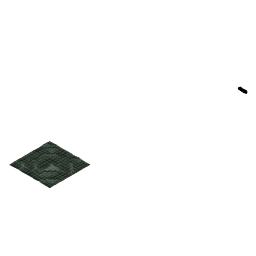
portal (Autodesk Fusion 360 design; units mm, degrees)
Autodesk Fusion 360 part; units mm, degrees
sketch "Sketch1" plane through (0, 0, 0) normal (0, 0, 1) x (1, 0, 0)
  line L0 (0, 0) -> (-55.5557, 0)
  line L1 (-55.5557, 0) -> (-55.5557, 55.5557)
  line L2 (-55.5557, 55.5557) -> (0, 55.5557)
  line L3 (0, 55.5557) -> (0, 0)
  line L4 (-55.5557, 55.5557) -> (0, 55.5557)
  line L5 (0, 55.5557) -> (0, 111.1113)
  line L6 (0, 111.1113) -> (-55.5557, 111.1113)
  line L7 (-55.5557, 111.1113) -> (-55.5557, 55.5557)
  line L8 (-55.5557, 111.1113) -> (0, 111.1113)
  line L9 (0, 111.1113) -> (0, 166.667)
  line L10 (0, 166.667) -> (-55.5557, 166.667)
  line L11 (-55.5557, 166.667) -> (-55.5557, 111.1113)
  line L12 (-55.5557, 166.667) -> (0, 166.667)
  line L13 (0, 166.667) -> (0, 222.2227)
  line L14 (0, 222.2227) -> (-55.5557, 222.2227)
  line L15 (-55.5557, 222.2227) -> (-55.5557, 166.667)
  line L16 (-55.5557, 0) -> (0, 0)
  line L17 (0, 0) -> (0, -55.5557)
  line L18 (0, -55.5557) -> (-55.5557, -55.5557)
  line L19 (-55.5557, -55.5557) -> (-55.5557, 0)
  line L20 (0, 0) -> (55.5557, 0)
  line L21 (55.5557, 0) -> (55.5557, -55.5557)
  line L22 (55.5557, -55.5557) -> (0, -55.5557)
  line L23 (0, -55.5557) -> (0, 0)
  line L24 (55.5557, 0) -> (111.1113, 0)
  line L25 (111.1113, 0) -> (111.1113, -55.5557)
  line L26 (111.1113, -55.5557) -> (55.5557, -55.5557)
  line L27 (55.5557, -55.5557) -> (55.5557, 0)
  line L28 (111.1113, -55.5557) -> (166.667, -55.5557)
  line L29 (166.667, -55.5557) -> (166.667, 0)
  line L30 (166.667, 0) -> (111.1113, 0)
  line L31 (111.1113, 0) -> (111.1113, -55.5557)
  line L32 (166.667, 0) -> (111.1113, 0)
  line L33 (111.1113, 0) -> (111.1113, 55.5557)
  line L34 (111.1113, 55.5557) -> (166.667, 55.5557)
  line L35 (166.667, 55.5557) -> (166.667, 0)
  line L36 (111.1113, 55.5557) -> (166.667, 55.5557)
  line L37 (166.667, 55.5557) -> (166.667, 111.1113)
  line L38 (166.667, 111.1113) -> (111.1113, 111.1113)
  line L39 (111.1113, 111.1113) -> (111.1113, 55.5557)
  line L40 (111.1113, 111.1113) -> (166.667, 111.1113)
  line L41 (166.667, 111.1113) -> (166.667, 166.667)
  line L42 (166.667, 166.667) -> (111.1113, 166.667)
  line L43 (111.1113, 166.667) -> (111.1113, 111.1113)
  line L44 (111.1113, 166.667) -> (166.667, 166.667)
  line L45 (166.667, 166.667) -> (166.667, 222.2227)
  line L46 (166.667, 222.2227) -> (111.1113, 222.2227)
  line L47 (111.1113, 222.2227) -> (111.1113, 166.667)
  line L48 (111.1113, 222.2227) -> (55.5557, 222.2227)
  line L49 (55.5557, 222.2227) -> (55.5557, 166.667)
  line L50 (55.5557, 166.667) -> (111.1113, 166.667)
  line L51 (111.1113, 166.667) -> (111.1113, 222.2227)
  line L52 (0, 222.2227) -> (55.5557, 222.2227)
  line L53 (55.5557, 222.2227) -> (55.5557, 166.667)
  line L54 (55.5557, 166.667) -> (0, 166.667)
  line L55 (0, 166.667) -> (0, 222.2227)
  dimension "d4" = 55.5557
  dimension "d5" = 55.5557
  dimension "d6" = 55.5557
  dimension "d7" = 55.5557
  dimension "d8" = 55.5557
  dimension "d9" = 55.5557
  dimension "d10" = 55.5557
  dimension "d11" = 55.5557
  dimension "d12" = 55.5557
  dimension "d13" = 55.5557
  dimension "d14" = 55.5557
  dimension "d15" = 55.5557
  dimension "d16" = 55.5557
  dimension "d17" = 55.5557
  dimension "d18" = 55.5557
  dimension "d19" = 55.5557
  dimension "d20" = 55.5557
  dimension "d21" = 55.5557
  dimension "d22" = 55.5557
  dimension "d23" = 55.5557
  dimension "d24" = 55.5557
  dimension "d25" = 55.5557
  dimension "d26" = 55.5557
  dimension "d27" = 55.5557
  dimension "d28" = 55.5557
  dimension "d29" = 55.5557
  dimension "d30" = 55.5557
  dimension "d31" = 55.5557
  constraint coincident L0.start L3.end
  constraint horizontal L0
  constraint vertical L1
  constraint horizontal L2
  constraint vertical L3
  constraint horizontal L4
  constraint vertical L5
  constraint horizontal L6
  constraint vertical L7
  constraint horizontal L8
  constraint vertical L9
  constraint horizontal L10
  constraint vertical L11
  constraint horizontal L12
  constraint vertical L13
  constraint horizontal L14
  constraint vertical L15
  constraint horizontal L16
  constraint vertical L17
  constraint horizontal L18
  constraint vertical L19
  constraint horizontal L20
  constraint vertical L21
  constraint horizontal L22
  constraint vertical L23
  constraint horizontal L24
  constraint vertical L25
  constraint horizontal L26
  constraint vertical L27
  constraint horizontal L28
  constraint vertical L29
  constraint horizontal L30
  constraint vertical L31
  constraint horizontal L32
  constraint vertical L33
  constraint horizontal L34
  constraint vertical L35
  constraint horizontal L36
  constraint vertical L37
  constraint horizontal L38
  constraint vertical L39
  constraint horizontal L40
  constraint vertical L41
  constraint horizontal L42
  constraint vertical L43
  constraint horizontal L44
  constraint vertical L45
  constraint horizontal L46
  constraint vertical L47
  constraint horizontal L48
  constraint vertical L49
  constraint horizontal L50
  constraint vertical L51
  constraint horizontal L52
  constraint vertical L53
  constraint horizontal L54
  constraint vertical L55
  measures "d4" distance of L0.start L0.end
  measures "d5" distance of L0.start L2.end
  measures "d6" distance of L1.end L2.end
  measures "d7" distance of L1.end L6.end
  measures "d8" distance of L6.end L5.end
  measures "d9" distance of L6.end L10.end
  measures "d10" distance of L10.end L9.end
  measures "d11" distance of L10.end L14.end
  measures "d12" distance of L0.end L0.start
  measures "d13" distance of L0.end L18.end
  measures "d14" distance of L0.start L20.end
  measures "d15" distance of L0.start L17.end
  measures "d16" distance of L20.end L24.end
  measures "d17" distance of L20.end L21.end
  measures "d18" distance of L25.end L28.end
  measures "d19" distance of L25.end L24.end
  measures "d20" distance of L29.end L24.end
  measures "d21" distance of L29.end L34.end
  measures "d22" distance of L33.end L34.end
  measures "d23" distance of L33.end L38.end
  measures "d24" distance of L38.end L37.end
  measures "d25" distance of L38.end L42.end
  measures "d26" distance of L42.end L41.end
  measures "d27" distance of L42.end L46.end
  measures "d28" distance of L46.end L48.end
  measures "d29" distance of L46.end L42.end
  measures "d30" distance of L13.end L48.end
  measures "d31" distance of L13.end L9.end
extrude "Extrude1" add sketch "Sketch1" along normal blind 30 contours L0 L16 L17 L18 L19 L23 | L0 L1 L2 L3 L4 L16 | L17 L20 L21 L22 L23 L27 | L2 L4 L5 L6 L7 L8 | L21 L24 L25 L26 L27 L31 | L6 L8 L9 L10 L11 L12 | L25 L28 L29 L30 L31 L32 | L30 L32 L33 L34 L35 L36 | L10 L12 L13 L14 L15 L55 | L13 L49 L52 L53 L54 L55 | L34 L36 L37 L38 L39 L40 | L47 L48 L49 L50 L51 L53 | L38 L40 L41 L42 L43 L44 | L42 L44 L45 L46 L47 L51 makes body 1
sketch "Sketch2" plane through (0, 0, 30) normal (0, 0, 1) x (-1, 0, 0)
  line L0 (0, -166.667) -> (-111.1113, -166.667)
  line L1 (-111.1113, -166.667) -> (-111.1113, 0)
  line L2 (-111.1113, 0) -> (0, 0)
  line L3 (0, 0) -> (0, -166.667)
  line L4 (55.5557, -222.2227) -> (55.5557, 55.5557)
  line L5 (55.5557, 55.5557) -> (-166.667, 55.5557)
  line L6 (-166.667, 55.5557) -> (-166.667, -222.2227)
  line L7 (-166.667, -222.2227) -> (55.5557, -222.2227)
  line L8 (50.5557, 50.5557) -> (-161.667, 50.5557)
  line L9 (-161.667, 50.5557) -> (-161.667, -217.2227)
  line L10 (-161.667, -217.2227) -> (50.5557, -217.2227)
  line L11 (50.5557, -217.2227) -> (50.5557, 50.5557)
  dimension "d34" = -5
extrude "Extrude2" cut sketch "Sketch2" against normal blind 25 contours L8 L9 L10 L11 bodies 1
sketch "Sketch3" plane through (0, 0, 5) normal (0, 0, 1) x (-1, 0, 0)
  line L0 (-111.1113, 0) -> (0, 0)
  line L1 (0, 0) -> (0, -166.667)
  line L2 (0, -166.667) -> (-111.1113, -166.667)
  line L3 (-111.1113, -166.667) -> (-111.1113, 0)
  line L4 (50.5557, -217.2227) -> (50.5557, 50.5557)
  line L5 (50.5557, 50.5557) -> (-161.667, 50.5557)
  line L6 (-161.667, 50.5557) -> (-161.667, -217.2227)
  line L7 (-161.667, -217.2227) -> (50.5557, -217.2227)
  line L8 (-118.1113, -173.667) -> (-118.1113, 7)
  line L9 (-118.1113, 7) -> (7, 7)
  line L10 (7, 7) -> (7, -173.667)
  line L11 (7, -173.667) -> (-118.1113, -173.667)
  line L12 (-121.1113, -176.667) -> (-121.1113, 10)
  line L13 (-121.1113, 10) -> (10, 10)
  line L14 (10, 10) -> (10, -176.667)
  line L15 (10, -176.667) -> (-121.1113, -176.667)
  dimension "d37" = -7
  dimension "d38" = -3
extrude "Extrude3" add sketch "Sketch3" along normal blind 15 separate body contours L12 L13 L14 L15 makes body 2
sketch "Sketch4" plane through (0, 0, 5) normal (0, 0, 1) x (-1, 0, 0)
  line L0 (-111.1113, 0) -> (0, 0)
  line L1 (0, 0) -> (0, -166.667)
  line L2 (0, -166.667) -> (-111.1113, -166.667)
  line L3 (-111.1113, -166.667) -> (-111.1113, 0)
  line L4 (50.5557, -217.2227) -> (50.5557, 50.5557)
  line L5 (50.5557, 50.5557) -> (-161.667, 50.5557)
  line L6 (-161.667, 50.5557) -> (-161.667, -217.2227)
  line L7 (-161.667, -217.2227) -> (50.5557, -217.2227)
  line L8 (23, 23) -> (23, -189.667)
  line L9 (23, -189.667) -> (-134.1113, -189.667)
  line L10 (-134.1113, -189.667) -> (-134.1113, 23)
  line L11 (-134.1113, 23) -> (23, 23)
  line L12 (26, -192.667) -> (-137.1113, -192.667)
  line L13 (-137.1113, -192.667) -> (-137.1113, 26)
  line L14 (-137.1113, 26) -> (26, 26)
  line L15 (26, 26) -> (26, -192.667)
  dimension "d41" = -23
  dimension "d42" = -3
extrude "Extrude4" add sketch "Sketch4" along normal blind 15 separate body contours L12 L13 L14 L15 makes body 3
sketch "Sketch5" plane through (134.1113, 0, 0) normal (-1, 0, 0) x (0, -1, 0)
  line L0 (-189.667, 5) -> (23, 5)
  line L1 (23, 5) -> (23, 20)
  line L2 (23, 20) -> (-189.667, 20)
  line L3 (-189.667, 20) -> (-189.667, 5)
sketch "Sketch6" plane through (0, 0, 20) normal (0, 0, 1) x (-1, 0, 0)
  line L0 (-134.1113, -189.667) -> (-134.1113, 23)
  line L1 (-134.1113, 23) -> (23, 23)
  line L2 (23, 23) -> (23, -189.667)
  line L3 (23, -189.667) -> (-134.1113, -189.667)
  line L4 (26, 26) -> (-137.1113, 26)
  line L5 (-137.1113, 26) -> (-137.1113, -192.667)
  line L6 (-137.1113, -192.667) -> (26, -192.667)
  line L7 (26, -192.667) -> (26, 26)
sketch "Sketch7" plane through (0, 0, 20) normal (0, 0, 1) x (-1, 0, 0)
  line L0 (7, 7) -> (7, -173.667)
  line L1 (7, -173.667) -> (-118.1113, -173.667)
  line L2 (-118.1113, -173.667) -> (-118.1113, 7)
  line L3 (-118.1113, 7) -> (7, 7)
  line L4 (10, -176.667) -> (10, 10)
  line L5 (10, 10) -> (-121.1113, 10)
  line L6 (-121.1113, 10) -> (-121.1113, -176.667)
  line L7 (-121.1113, -176.667) -> (10, -176.667)
  line L8 (-118.1113, -173.667) -> (-113.1113, -173.667)
  line L9 (-113.1113, -173.667) -> (-113.1113, -176.667)
  line L10 (-113.1113, -176.667) -> (-118.1113, -176.667)
  line L11 (-118.1113, -176.667) -> (-118.1113, -173.667)
  dimension "d45" = 5
  constraint horizontal L8
  constraint vertical L9
  constraint horizontal L10
  constraint vertical L11
  constraint coincident L1.end L2.start
  measures "d45" distance of L1.end L8.end
sketch "Sketch8" plane through (0, 0, 20) normal (0, 0, 1) x (-1, 0, 0)
  line L0 (-134.1113, -189.667) -> (-134.1113, 23)
  line L1 (-134.1113, 23) -> (23, 23)
  line L2 (23, 23) -> (23, -189.667)
  line L3 (23, -189.667) -> (-134.1113, -189.667)
  line L4 (26, 26) -> (-137.1113, 26)
  line L5 (-137.1113, 26) -> (-137.1113, -192.667)
  line L6 (-137.1113, -192.667) -> (26, -192.667)
  line L7 (26, -192.667) -> (26, 26)
  line L8 (-134.1113, -189.667) -> (-128.1113, -189.667)
  line L9 (-128.1113, -189.667) -> (-128.1113, -192.667)
  line L10 (-128.1113, -192.667) -> (-134.1113, -192.667)
  line L11 (-134.1113, -192.667) -> (-134.1113, -189.667)
  dimension "d46" = 6
  dimension "d47" = 3
  constraint horizontal L8
  constraint vertical L9
  constraint horizontal L10
  constraint vertical L11
  constraint coincident L0.start L3.end
  measures "d46" distance of L0.start L8.end
  measures "d47" distance of L0.start L10.end
extrude "Extrude5" cut sketch "Sketch8" against normal blind 15 contours L3 L6 L8 L9 L10 L11 bodies 3
sketch "Sketch9" plane through (0, 217.2227, 0) normal (0, -1, 0) x (1, 0, 0)
  line L0 (161.667, 30) -> (-50.5557, 30)
  line L1 (-50.5557, 30) -> (-50.5557, 5)
  line L2 (-50.5557, 5) -> (161.667, 5)
  line L3 (161.667, 5) -> (161.667, 30)
  line L4 (105, 15) -> (105, 29)
  line L5 (93, 29) -> (93, 15)
  line L6 (93, 15) -> (105, 15)
  line L7 (93, 29) -> (93, 30)
  line L8 (93, 30) -> (105, 30)
  line L9 (105, 30) -> (105, 29)
  constraint vertical L4
  constraint perpendicular L4 L6
  constraint vertical L7
  constraint horizontal L8
  constraint vertical L9
  constraint coincident L0 L7.end
extrude "Extrude6" cut sketch "Sketch9" against normal blind 2 contours L0 L4 L5 L6 L7 L8 L9 bodies 1
sketch "Sketch10" plane through (0, 219.2227, 0) normal (0, -1, 0) x (1, 0, 0)
  line L0 (93, 30) -> (93, 15)
  line L1 (93, 15) -> (105, 15)
  line L2 (105, 15) -> (105, 30)
  line L3 (105, 30) -> (93, 30)
  line L4 (105, 15) -> (93, 15)
  line L5 (93, 15) -> (93, 30)
  line L6 (93, 30) -> (105, 30)
  line L7 (105, 30) -> (105, 15)
  constraint horizontal L4
  constraint vertical L5
  constraint horizontal L6
  constraint vertical L7
  constraint coincident L0.start L3.end
  constraint coincident L1.end L2.start
extrude "Extrude7" add sketch "Sketch10" along normal blind 2 separate body makes body 4
sketch "Sketch11" plane through (0, 217.2227, 0) normal (0, -1, 0) x (1, 0, 0)
  line L0 (105, 30) -> (93, 30)
  line L1 (93, 30) -> (93, 15)
  line L2 (93, 15) -> (105, 15)
  line L3 (105, 15) -> (105, 30)
sketch "Sketch12" plane through (0, 217.2227, 0) normal (0, -1, 0) x (1, 0, 0)
  line L0 (105, 30) -> (93, 30)
  line L1 (93, 30) -> (93, 15)
  line L2 (93, 15) -> (105, 15)
  line L3 (105, 15) -> (105, 30)
  circle A0 centre (102.56, 17.44) radius 0.75
  circle A1 centre (100.12, 17.44) radius 0.75
  circle A2 centre (97.68, 17.44) radius 0.75
  circle A3 centre (95.24, 17.44) radius 0.75
  dimension "d56" = 2.44
  dimension "d57" = 2.44
  dimension "d58" = 2.44
  dimension "d59" = 1.5
  dimension "d60" = 1.5
  dimension "d61" = 1.5
  dimension "d62" = 1.5
  measures "d56" distance of A0.centre A1.centre
  measures "d57" distance of A1.centre A2.centre
  measures "d58" distance of A2.centre A3.centre
  measures "d59" diameter of A0
  measures "d60" diameter of A1
  measures "d61" diameter of A2
  measures "d62" diameter of A3
extrude "Extrude8" cut sketch "Sketch12" against normal blind 85 contours A0 bodies 4
extrude "Extrude9" cut sketch "Sketch12" against normal blind 9 contours A1 bodies 4
extrude "Extrude10" cut sketch "Sketch12" against normal blind 5 contours A2 bodies 4
extrude "Extrude11" cut sketch "Sketch12" against normal blind 9 contours A3 bodies 4
sketch "Sketch13" plane through (0, 0, 30) normal (0, 0, 1) x (-1, 0, 0)
  line L0 (-105, -219.2227) -> (-93, -219.2227)
  line L1 (-93, -219.2227) -> (-93, -217.2227)
  line L2 (-93, -217.2227) -> (-105, -217.2227)
  line L3 (-105, -217.2227) -> (-105, -219.2227)
  line L4 (-99, -217.2227) -> (-99, -219.2227) construction
  line L5 (-94, -217.4727) -> (-104, -217.4727)
  line L6 (-104, -217.4727) -> (-104, -218.9727)
  line L7 (-104, -218.9727) -> (-94, -218.9727)
  line L8 (-94, -218.9727) -> (-94, -217.4727)
  line L9 (-94, -217.4727) -> (-104, -218.9727) construction
  line L10 (-104, -217.4727) -> (-94, -218.9727) construction
  point P0 (-99, -218.2227)
  dimension "d71" = 10
  dimension "d72" = 1.5
  constraint midpoint L2 L4.start
  constraint midpoint L0 L4.end
  constraint horizontal L5
  constraint perpendicular L5 L6
  constraint parallel L5 L7
  constraint parallel L6 L8
  constraint coincident L9 P0
  constraint coincident L10 P0
  constraint midpoint L4 P0
  measures "d71" distance of L6.end L7.end
  measures "d72" distance of L5.end L6.end
extrude "Extrude12" add sketch "Sketch13" along normal blind 2 separate body contours L5 L6 L7 L8 makes body 5
move_body "Move1" bodies 5 to x (1, 0, 0) y (0, 1, 0) z (0, 0, 1) at (0, -1.7, -2.1)
sketch "Sketch14" plane through (0, 0, 5) normal (0, 0, 1) x (-1, 0, 0)
  line L0 (-111.1113, 0) -> (0, 0)
  line L1 (0, 0) -> (0, -166.667)
  line L2 (0, -166.667) -> (-111.1113, -166.667)
  line L3 (-111.1113, -166.667) -> (-111.1113, 0)
  line L4 (50.5557, -217.2227) -> (50.5557, 50.5557)
  line L5 (50.5557, 50.5557) -> (-161.667, 50.5557)
  line L6 (-161.667, 50.5557) -> (-161.667, -217.2227)
  line L7 (-161.667, -217.2227) -> (50.5557, -217.2227)
sketch "Sketch15" plane through (0, -50.5557, 0) normal (0, 1, 0) x (-1, 0, 0)
  line L0 (50.5557, 30) -> (-161.667, 30)
  line L1 (-161.667, 30) -> (-161.667, 5)
  line L2 (-161.667, 5) -> (50.5557, 5)
  line L3 (50.5557, 5) -> (50.5557, 30)
extrude "Extrude13" add 1 faces at (-53.889, 38.7038, 30) along direction (0, 0, 1) blind 5 on bodies 1 bodies 1 4
sketch "Sketch16" plane through (0, -50.5557, 0) normal (0, 1, 0) x (-1, 0, 0)
  line L0 (-161.667, 35) -> (-161.667, 5)
  line L1 (-161.667, 5) -> (50.5557, 5)
  line L2 (50.5557, 5) -> (50.5557, 35)
  line L3 (50.5557, 35) -> (-161.667, 35)
fillet "Fillet1" radius 15 13 edges at (118.1113, -7, 12.5) (-7, -7, 12.5) (-10, -10, 12.5) (121.1113, -10, 12.5) (-7, 173.667, 12.5) (121.1113, 176.667, 12.5) (118.1113, 173.667, 12.5) (134.1113, -23, 12.5) (-23, -23, 12.5) (-26, -26, 12.5) (137.1113, -26, 12.5) (-23, 189.667, 12.5) (-26, 192.667, 12.5) on bodies 2 3
fillet "Fillet2" radius 15 1 edges at (-10, 176.667, 12.5) on bodies 2
fillet "Fillet3" radius 1 4 edges at (134.1113, 192.667, 12.5) (137.1113, 192.667, 12.5) (128.1113, 192.667, 12.5) (128.1113, 189.667, 12.5) on bodies 3
sketch "Sketch17" plane through (0, 0, 35) normal (0, 0, 1) x (-1, 0, 0)
  line L0 (55.5557, -222.2227) -> (55.5557, 55.5557)
  line L1 (55.5557, 55.5557) -> (-166.667, 55.5557)
  line L2 (-166.667, 55.5557) -> (-166.667, -222.2227)
  line L3 (-166.667, -222.2227) -> (55.5557, -222.2227)
  line L4 (-93, -217.2227) -> (-93, -219.2227)
  line L5 (-93, -219.2227) -> (-105, -219.2227)
  line L6 (-105, -219.2227) -> (-105, -217.2227)
  line L7 (-105, -217.2227) -> (-161.667, -217.2227)
  line L8 (-161.667, -217.2227) -> (-161.667, 50.5557)
  line L9 (-161.667, 50.5557) -> (50.5557, 50.5557)
  line L10 (50.5557, 50.5557) -> (50.5557, -217.2227)
  line L11 (50.5557, -217.2227) -> (-93, -217.2227)
sketch "Sketch18" plane through (0, 0, 0) normal (0, 1, 0) x (1, 0, 0)
sketch "Sketch19" plane through (0, 0, 0) normal (1, 0, 0) x (0, 1, 0)
sketch "Sketch20" plane through (0, 0, 0) normal (0, 0, 1) x (1, 0, 0)
  line L0 (55, 0) -> (0, 0)
  line L1 (0, 0) -> (0, 55)
  line L2 (0, 55) -> (55, 55)
  line L3 (55, 55) -> (55, 0)
  constraint horizontal L0
  constraint vertical L1
  constraint horizontal L2
  constraint vertical L3
other "Base Mesh Feature3"
other "MeshReduce1"
extrude "Extrude14" add sketch "Sketch20" along normal blind 3 separate body makes body 6
hidden bodies 1 2 3 6
equation "d4 = 166.667 mm / 3"
equation "d5 = 166.667 mm / 3"
equation "d6 = 166.667 mm / 3"
equation "d7 = 166.667 mm / 3"
equation "d8 = 166.667 mm / 3"
equation "d9 = 166.667 mm / 3"
equation "d10 = 166.667 mm / 3"
equation "d11 = 166.667 mm / 3"
equation "d12 = 166.667 mm / 3"
equation "d13 = 166.667 mm / 3"
equation "d14 = 166.667 mm / 3"
equation "d15 = 166.667 mm / 3"
equation "d16 = 166.667 mm / 3"
equation "d17 = 166.667 mm / 3"
equation "d18 = 166.667 mm / 3"
equation "d19 = 166.667 mm / 3"
equation "d20 = 166.667 mm / 3"
equation "d21 = 166.667 mm / 3"
equation "d22 = 166.667 mm / 3"
equation "d23 = 166.667 mm / 3"
equation "d24 = 166.667 mm / 3"
equation "d25 = 166.667 mm / 3"
equation "d26 = 166.667 mm / 3"
equation "d27 = 166.667 mm / 3"
equation "d28 = 166.667 mm / 3"
equation "d29 = 166.667 mm / 3"
equation "d30 = 166.667 mm / 3"
equation "d31 = 166.667 mm / 3"
named bodies: "outer shell", "white led diffuser", "led wall"
